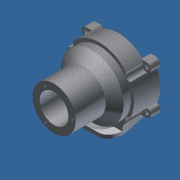
# Autodesk Inventor part: Drill Mtl Housing Dewalt XRP
Saved by Autodesk Inventor 2012 (Build 160160000, 160)
## iProperties
Created: 2012-07-04
Part Number: Drill Mtl Housing Dewalt XRP
Material: Default
Document SubType Name: Modeling
Designer: Bruce
Density: 1 g/cm^3
Author: Bruce
Autodesk Inventor part; units mm, degrees
ref_plane "XZ Plane" through (0, 0, 0) normal (0, 1, 0) x (-1, 0, 0)
ref_plane "XY Plane" through (0, 0, 0) normal (0, 0, 1) x (1, 0, 0)
sketch "Sketch1" plane through (0, 0, 0) normal (0, 0, 1) x (1, 0, 0)
  circle A0 centre (0, 0) radius 19.05
  circle A1 centre (0, 0) radius 15.875 construction
  circle A2 centre (-8.255, 13.5599) radius 1.6256
  circle A3 centre (-7.6157, -13.929) radius 1.6256
  circle A4 centre (15.8707, 0.3691) radius 1.6256
  circle A5 centre (0, 0) radius 12.7
  dimension "d1" = 31.75
  dimension "d0" = 38.1
  dimension "d2" = 8.255
  dimension "d3" = 3.2512
  dimension "d6" = 360
  dimension "d8" = 25.4
  constraints: 5 centre point, 3 coincident, 10 other
  measures "d0" diameter of A0
  measures "d2" horizontal distance of A2.centre point (0, 0)
  measures "d3" diameter of A2
  measures "d8" diameter of A5
extrude "Extrusion1" add sketch "Sketch1" against normal blind 24.892
thread "Thread1" size "6-32 UNC" class "2B" standard "ANSI Unified Screw Threads" full length
thread "Thread2" size "6-32 UNC" class "2B" standard "ANSI Unified Screw Threads" full length
thread "Thread3" size "6-32 UNC" class "2B" standard "ANSI Unified Screw Threads" full length
sketch "Sketch3" plane through (0, 0, 0) normal (1, 0, 0) x (0, 1, 0)
  line L0 (19.05, -24.892) -> (-19.05, -24.892) projected
  line L1 (19.05, 0) -> (19.05, -24.892) projected
  line L2 (19.05, -24.892) -> (-19.05, -24.892) projected
  line L3 (-19.05, 0) -> (19.05, 0) projected
  line L4 (-19.05, 0) -> (-19.05, -24.892) projected
  line L5 (-19.05, 0) -> (19.05, 0) projected
  line L6 (-19.05, 0) -> (-19.05, -24.892) projected
  line L7 (19.05, 0) -> (19.05, -24.892) projected
  line L8 (0, -24.892) -> (19.05, -24.892)
  line L9 (27.6225, -40.132) -> (0, -40.132)
  line L10 (0, -40.132) -> (0, -24.892)
  line L11 (27.6225, -33.782) -> (19.05, -26.4795)
  line L12 (19.05, -26.4795) -> (19.05, -24.892)
  line L13 (27.6225, -33.782) -> (27.6225, -40.132)
  line L14 (0, -40.132) -> (30.48, -40.132)
  line L15 (30.48, -40.132) -> (30.48, -63.5)
  line L16 (30.48, -63.5) -> (0, -63.5)
  line L17 (0, -63.5) -> (0, -40.132)
  point P0 (0, 0)
  dimension "d17" = 38.1
  dimension "d18" = 27.6225
  dimension "d19" = 6.35
  dimension "d20" = 1.5875
  dimension "d21" = 30.48
  dimension "d23" = 15.24
  dimension "d24" = 63.5
  constraints: 20 end point, 4 parallel, 2 horizontal, 2 perpendicular, 1 collinear, 1 midpoint
  measures "d17" distance between parallel lines of L4 L1
  measures "d18" distance of L9.start L9.end
  measures "d19" distance of L11.start L9.start
  measures "d20" distance of L11.end L7.end
  measures "d21" distance of L15.end L16.end
  measures "d23" distance of L9.end L8.start
  measures "d24" distance between parallel lines of L16 L5
revolve "Revolution1" add sketch "Sketch3" angle 360 about axis through (0, 0, -63.5) along (0, 0, 1) contours L12 L11 L13 L9 L10 L0 | L9 L14 L15 L16 L17
sketch "Sketch4" plane through (0, 0, -63.5) normal (0, 0, -1) x (-1, 0, 0)
  circle A0 centre (0, 0) radius 30.48 projected
  circle A1 centre (0, 0) radius 31.9786 construction
  arc A2 (-23.5091, 19.3998) -> (-27.2381, 13.679) centre (-26.7898, 17.4625) ccw
  circle A3 centre (-26.7898, 17.4625) radius 1.7018
  line L0 (-26.7898, 21.2725) -> (-21.8291, 21.2725)
  arc A4 (-21.8291, 21.2725) -> (-23.5091, -19.3998) centre (0, 0) ccw
  arc A5 (28.6765, 14.1524) -> (27.2381, 13.679) centre (26.7898, 17.4625) ccw
  circle A6 centre (26.7898, 17.4625) radius 1.7018
  line L1 (26.7898, 21.2725) -> (21.8291, 21.2725)
  arc A7 (-27.2381, -13.679) -> (-23.5091, -19.3998) centre (-26.7898, -17.4625) ccw
  circle A8 centre (-26.7898, -17.4625) radius 1.7018
  circle A9 centre (26.7898, -17.4625) radius 1.7018
  arc A10 (24.5228, -20.5247) -> (27.2381, -13.679) centre (26.7898, -17.4625) ccw
  line L2 (-26.7898, -21.2725) -> (-21.8291, -21.2725)
  line L3 (26.7898, -21.2725) -> (21.8291, -21.2725)
  arc A11 (18.7731, 18.2943) -> (-18.7731, 18.2943) centre (0, 0) ccw
  arc A12 (20.7832, 20.2532) -> (-20.7832, 20.2532) centre (0, 0) ccw
  arc A13 (-18.7731, 18.2943) -> (-18.7731, -18.2943) centre (0, 0) ccw
  arc A14 (-18.7731, -18.2943) -> (18.7731, 18.2943) centre (0, 0) ccw
  line L4 (-18.7731, 18.2943) -> (-21.8291, 21.2725)
  line L5 (18.7731, 18.2943) -> (21.8291, 21.2725)
  arc A15 (-27.2381, 13.679) -> (-23.5091, 19.3998) centre (-26.7898, 17.4625) ccw
  arc A16 (21.8291, 21.2725) -> (-21.8291, 21.2725) centre (0, 0) ccw
  arc A17 (23.5091, 19.3998) -> (21.8291, 21.2725) centre (0, 0) ccw
  arc A18 (-23.5091, -19.3998) -> (23.5091, 19.3998) centre (0, 0) ccw
  arc A19 (23.5091, -19.3998) -> (24.5228, -20.5247) centre (26.7898, -17.4625) ccw
  arc A20 (-23.5091, -19.3998) -> (-27.2381, -13.679) centre (-26.7898, -17.4625) ccw
  arc A21 (27.2381, -13.679) -> (23.5091, -19.3998) centre (26.7898, -17.4625) ccw
  arc A22 (27.2381, 13.679) -> (28.6765, 14.1524) centre (26.7898, 17.4625) ccw
  point P0 (-24.3095, 21.2725)
  dimension "d26" = 63.9572
  dimension "d27" = 7.62
  dimension "d28" = 3.4036
  dimension "d29" = 17.4625
  dimension "d30" = 7.62
  dimension "d31" = 3.4036
  dimension "d32" = 7.62
  dimension "d33" = 3.4036
  dimension "d34" = 7.62
  dimension "d35" = 3.4036
  dimension "d36" = 60.96
  dimension "d37" = 52.4256
  dimension "d38" = 1.4605
  dimension "d66" = 26.7898
  constraints: 57 point on circle, 21 centre point, 12 end point, 8 coincident, 5 tangent, 4 horizontal, 2 point on line, 2 vertical alignment, 1 concentric, 1 horizontal alignment, 1 midpoint, 11 other
  measures "d26" diameter of A1
  measures "d27" diameter of A2
  measures "d28" diameter of A3
  measures "d29" vertical distance of A0.centre A1.start
  measures "d30" diameter of A5
  measures "d31" diameter of A6
  measures "d32" diameter of A7
  measures "d33" diameter of A8
  measures "d34" diameter of A10
  measures "d35" diameter of A9
  measures "d36" diameter of A0
  measures "d37" diameter of A11
  measures "d38" radial gap between concentric circles of A12 A0
  measures "d66" horizontal distance of A1.start A0.centre
extrude "Extrusion2" add sketch "Sketch4" against normal blind 8.509 contours A0 A6 A5 A22 | A10 A19 A0 A9 | A0 A6 | A0 L1 A5 | A9 A0 | L3 A0 A19 A10 | A0 A2 L0 | L2 A7 A0 | A0 A3 A2 | A7 A0 A8 | A0 A3 | A8 A0 picked at (26.4505, 17.1876) picked at (26.4505, -17.1876) picked at (-26.4025, 17.2615) picked at (-26.4025, -17.2615)
extrude "Extrusion3" cut sketch "Sketch4" against normal through all contours A6 A0 | A0 A6 | A9 A0 | A0 A9 | A3 A0 | A0 A3 | A8 A0 | A0 A8
extrude "Extrusion4" cut sketch "Sketch4" against normal blind 25.4 contours A14 A13 A11
extrude "Extrusion5" cut sketch "Sketch4" against normal blind 19.05 contours L5 A12 L4 A0
extrude "Extrusion6" cut sketch "Sketch4" against normal blind 6.35 contours L5 A11 L4 A12
sketch "Sketch5" plane through (0, 0, -54.991) normal (0, 0, 1) x (1, 0, 0)
  arc A0 (-25.0959, 17.2981) -> (-25.9557, 15.9791) centre (-26.7898, 17.4625) ccw projected
  arc A1 (25.0959, -17.2981) -> (25.9557, -15.9791) centre (26.7898, -17.4625) ccw projected
  arc A2 (-25.9557, -15.9791) -> (-25.0959, -17.2981) centre (-26.7898, -17.4625) ccw projected
  arc A3 (-25.9557, 15.9791) -> (-25.9557, -15.9791) centre (0, 0) ccw projected
  arc A4 (25.0959, 17.2981) -> (-25.0959, 17.2981) centre (0, 0) ccw projected
  circle A5 centre (0, 0) radius 27.6225 projected
  arc A6 (-25.9557, 15.9791) -> (-25.0959, 17.2981) centre (-26.7898, 17.4625) ccw projected
  arc A7 (-25.9557, 15.9791) -> (-25.9557, -15.9791) centre (0, 0) ccw projected
  arc A8 (-25.0959, -17.2981) -> (-25.9557, -15.9791) centre (-26.7898, -17.4625) ccw projected
  arc A9 (-25.0959, -17.2981) -> (25.0959, -17.2981) centre (0, 0) ccw projected
  arc A10 (25.9557, -15.9791) -> (25.0959, -17.2981) centre (26.7898, -17.4625) ccw projected
  arc A11 (25.9557, -15.9791) -> (25.9557, 15.9791) centre (0, 0) ccw projected
  arc A12 (25.0959, 17.2981) -> (25.9557, 15.9791) centre (26.7898, 17.4625) ccw projected
  arc A13 (25.0959, 17.2981) -> (-25.0959, 17.2981) centre (0, 0) ccw projected
  arc A14 (25.0959, -17.2981) -> (25.9557, -15.9791) centre (26.7898, -17.4625) ccw projected
  arc A15 (21.8291, -21.2725) -> (25.0959, -17.2981) centre (0, 0) ccw projected
  line L0 (26.7898, -21.2725) -> (21.8291, -21.2725) projected
  arc A16 (26.7898, -21.2725) -> (27.2381, -13.679) centre (26.7898, -17.4625) ccw projected
  arc A17 (25.9557, -15.9791) -> (27.2381, -13.679) centre (0, 0) ccw projected
  arc A18 (-25.0959, 17.2981) -> (-25.9557, 15.9791) centre (-26.7898, 17.4625) ccw projected
  arc A19 (-21.8291, 21.2725) -> (-25.0959, 17.2981) centre (0, 0) ccw projected
  line L1 (-26.7898, 21.2725) -> (-21.8291, 21.2725) projected
  arc A20 (-26.7898, 21.2725) -> (-27.2381, 13.679) centre (-26.7898, 17.4625) ccw projected
  arc A21 (-25.9557, 15.9791) -> (-27.2381, 13.679) centre (0, 0) ccw projected
  arc A22 (-25.9557, -15.9791) -> (-25.0959, -17.2981) centre (-26.7898, -17.4625) ccw projected
  arc A23 (-27.2381, -13.679) -> (-25.9557, -15.9791) centre (0, 0) ccw projected
  arc A24 (-27.2381, -13.679) -> (-26.7898, -21.2725) centre (-26.7898, -17.4625) ccw projected
  line L2 (-21.8291, -21.2725) -> (-26.7898, -21.2725) projected
  arc A25 (-25.0959, -17.2981) -> (-21.8291, -21.2725) centre (0, 0) ccw projected
  circle A26 centre (-26.7898, 17.4625) radius 3.81
  circle A27 centre (26.7898, 17.4625) radius 3.81
  circle A28 centre (26.7898, -17.4625) radius 3.81
  circle A29 centre (-26.7898, -17.4625) radius 3.81
  constraints: 4 coincident, 3 centre point, 1 concentric, 1 tangent, 3 other
extrude "Extrusion7" cut sketch "Sketch5" along normal blind 25.4 contours A6 A0 | A0 A3 A20 A26 A4 | A4 A26 A3 A6 | A29 A9 A8 A3 | A3 A2 A9 A29 A24 | A27 A11 A12 A4 | A4 A12 A11 A27 | A8 A2 | A16 A28 A9 A1 A11 | A11 A10 A9 A28 | A1 A10
sketch "Sketch6" plane through (26.7898, -21.2725, -63.5) normal (0, 0, -1) x (-1, 0, 0)
  arc A0 (-0.4484, 34.9515) -> (-0.4484, 7.5935) centre (26.7898, 21.2725) ccw projected
  line L0 (53.5795, 42.545) -> (48.6189, 42.545) projected
  arc A1 (8.0167, 39.5669) -> (45.5628, 39.5669) centre (26.7898, 21.2725) ccw projected
  line L1 (7.2635, -12.7) -> (46.316, -12.7)
  line L2 (46.316, -12.7) -> (48.6189, 0)
  line L3 (7.2635, -12.7) -> (4.9606, 0)
  arc A2 (4.9606, 0) -> (48.6189, 0) centre (26.7898, 21.2725) ccw
  line L4 (0, 0) -> (4.9606, 0) projected
  dimension "d52" = 39.0525
  dimension "d53" = 19.5263
  dimension "d64" = 12.7
  constraints: 6 end point, 2 point on circle, 1 centre point, 1 coincident, 1 parallel
  measures "d52" distance of L1.start L1.end
  measures "d53" horizontal distance of L1.start A0.centre
  measures "d64" distance between parallel lines of L1 L4
extrude "Extrusion8" add sketch "Sketch6" against normal blind 31.75
ref_plane "Work Plane1" through (25.4, 0, 0) normal (1, 0, 0) x (0, 1, 0)
sketch "Sketch8" plane through (25.4, 0, 0) normal (1, 0, 0) x (0, 1, 0)
  line L0 (-21.2725, -31.75) -> (-33.9725, -31.75) projected
  line L1 (-33.9725, -63.5) -> (-33.9725, -31.75) projected
  line L2 (-21.2725, -63.5) -> (-33.9725, -63.5) projected
  line L3 (-21.2725, -63.5) -> (-21.2725, -54.991) projected
  line L4 (-21.2725, -40.132) -> (-21.2725, -54.991) projected
  line L5 (-21.2725, -40.132) -> (-21.2725, -31.75) projected
  line L6 (-27.6225, -33.782) -> (-27.6225, -40.132) projected
  line L7 (-27.6225, -33.782) -> (27.6225, -33.782) projected
  line L8 (-19.05, -26.4795) -> (19.05, -26.4795) projected
  line L9 (-19.05, -26.4795) -> (-27.6225, -33.782) projected
  line L10 (-21.2725, -63.5) -> (-21.2725, -54.991) projected
  line L11 (-22.86, -63.5) -> (-31.0388, -40.132)
  line L12 (-30.48, -40.132) -> (-21.2725, -40.132) projected
  line L13 (-33.9725, -31.75) -> (-33.9725, -63.5)
  line L14 (-22.86, -63.5) -> (-33.9725, -63.5)
  line L15 (-27.6225, -40.132) -> (-31.0388, -40.132)
  line L16 (-27.6225, -40.132) -> (-29.3346, -35.2404)
  line L17 (-30.5562, -31.75) -> (-33.9725, -31.75)
  line L18 (-21.2725, -40.132) -> (-27.6225, -40.132)
  line L19 (-21.2725, -40.132) -> (-21.2725, -31.75)
  line L20 (-30.5562, -31.75) -> (-21.2725, -31.75)
  line L21 (-29.3346, -35.2404) -> (-30.5562, -31.75)
  line L22 (-31.0388, -40.132) -> (-33.9725, -31.75)
  point P0 (0, 0)
  dimension "d58" = 1.5875
  constraints: 22 end point, 7 parallel, 3 perpendicular, 3 point on line, 1 collinear
  measures "d58" distance from line of L11.start L3
extrude "Extrusion9" cut sketch "Sketch8" against normal through all contours L22 L11 L2 L1
extrude "Extrusion10" cut sketch "Sketch8" against normal up to next contours L0 L9 L6 L16 L21 | L0 L5 L7 L9 | L7 L5 L12 L6
fillet "Fillet1" radius 12.7 2 edges at (19.836, -32.2644, -31.75) (-19.836, -32.2644, -31.75)
equation "\"d30\" = d27"
equation "\"d31\" = d28"
equation "\"d32\" = d27"
equation "\"d33\" = d28"
equation "\"d34\" = d27"
equation "\"d35\" = d28"
equation "\"d53\" = 0.5 * d52"
body "Solid1"
